Autodesk Fusion 360 part; units mm, degrees
(part 6 of 12)
  line L935 (-33.2373, 77.1244) -> (-33.2373, 72.1244)
  line L936 (-33.2373, 72.1244) -> (-28.9072, 69.6244)
  line L937 (-28.9072, 69.6244) -> (-24.577, 72.1244)
  line L938 (-24.577, 72.1244) -> (-24.577, 77.1244)
  line L939 (-24.577, 77.1244) -> (-28.9072, 79.6244)
  line L940 (-18.2469, 79.6244) -> (-22.577, 77.1244)
  line L941 (-22.577, 77.1244) -> (-22.577, 72.1244)
  line L942 (-22.577, 72.1244) -> (-18.2469, 69.6244)
  line L943 (-18.2469, 69.6244) -> (-13.9168, 72.1244)
  line L944 (-13.9168, 72.1244) -> (-13.9168, 77.1244)
  line L945 (-13.9168, 77.1244) -> (-18.2469, 79.6244)
  line L946 (-7.5866, 79.6244) -> (-11.9168, 77.1244)
  line L947 (-11.9168, 77.1244) -> (-11.9168, 72.1244)
  line L948 (-11.9168, 72.1244) -> (-7.5866, 69.6244)
  line L949 (-7.5866, 69.6244) -> (-3.2565, 72.1244)
  line L950 (-3.2565, 72.1244) -> (-3.2565, 77.1244)
  line L951 (-3.2565, 77.1244) -> (-7.5866, 79.6244)
  line L952 (3.0736, 79.6244) -> (-1.2565, 77.1244)
  line L953 (-1.2565, 77.1244) -> (-1.2565, 72.1244)
  line L954 (-1.2565, 72.1244) -> (3.0736, 69.6244)
  line L955 (3.0736, 69.6244) -> (7.4037, 72.1244)
  line L956 (7.4037, 72.1244) -> (7.4037, 77.1244)
  line L957 (7.4037, 77.1244) -> (3.0736, 79.6244)
  line L958 (13.7339, 79.6244) -> (9.4037, 77.1244)
  line L959 (9.4037, 77.1244) -> (9.4037, 72.1244)
  line L960 (9.4037, 72.1244) -> (13.7339, 69.6244)
  line L961 (13.7339, 69.6244) -> (18.064, 72.1244)
  line L962 (18.064, 72.1244) -> (18.064, 77.1244)
  line L963 (18.064, 77.1244) -> (13.7339, 79.6244)
  line L964 (24.3941, 79.6244) -> (20.064, 77.1244)
  line L965 (20.064, 77.1244) -> (20.064, 72.1244)
  line L966 (20.064, 72.1244) -> (24.3941, 69.6244)
  line L967 (24.3941, 69.6244) -> (28.7242, 72.1244)
  line L968 (28.7242, 72.1244) -> (28.7242, 77.1244)
  line L969 (28.7242, 77.1244) -> (24.3941, 79.6244)
  line L970 (35.0544, 79.6244) -> (30.7242, 77.1244)
  line L971 (30.7242, 77.1244) -> (30.7242, 72.1244)
  line L972 (30.7242, 72.1244) -> (35.0544, 69.6244)
  line L973 (35.0544, 69.6244) -> (39.3845, 72.1244)
  line L974 (39.3845, 72.1244) -> (39.3845, 77.1244)
  line L975 (39.3845, 77.1244) -> (35.0544, 79.6244)
  line L976 (45.7146, 79.6244) -> (41.3845, 77.1244)
  line L977 (41.3845, 77.1244) -> (41.3845, 72.1244)
  line L978 (41.3845, 72.1244) -> (45.7146, 69.6244)
  line L979 (45.7146, 69.6244) -> (50.0447, 72.1244)
  line L980 (50.0447, 72.1244) -> (50.0447, 77.1244)
  line L981 (50.0447, 77.1244) -> (45.7146, 79.6244)
  line L982 (56.3749, 79.6244) -> (52.0447, 77.1244)
  line L983 (52.0447, 77.1244) -> (52.0447, 72.1244)
  line L984 (52.0447, 72.1244) -> (56.3749, 69.6244)
  line L985 (56.3749, 69.6244) -> (60.705, 72.1244)
  line L986 (60.705, 72.1244) -> (60.705, 77.1244)
  line L987 (60.705, 77.1244) -> (56.3749, 79.6244)
  line L988 (-151.5001, 88.8564) -> (-155.8302, 86.3564)
  line L989 (-155.8302, 86.3564) -> (-155.8302, 81.3564)
  line L990 (-155.8302, 81.3564) -> (-151.5001, 78.8564)
  line L991 (-151.5001, 78.8564) -> (-147.17, 81.3564)
  line L992 (-147.17, 81.3564) -> (-147.17, 86.3564)
  line L993 (-147.17, 86.3564) -> (-151.5001, 88.8564)
  line L994 (-140.8398, 88.8564) -> (-145.17, 86.3564)
  line L995 (-145.17, 86.3564) -> (-145.17, 81.3564)
  line L996 (-145.17, 81.3564) -> (-140.8398, 78.8564)
  line L997 (-140.8398, 78.8564) -> (-136.5097, 81.3564)
  line L998 (-136.5097, 81.3564) -> (-136.5097, 86.3564)
  line L999 (-136.5097, 86.3564) -> (-140.8398, 88.8564)
  line L1000 (-130.1796, 88.8564) -> (-134.5097, 86.3564)
  line L1001 (-134.5097, 86.3564) -> (-134.5097, 81.3564)
  line L1002 (-134.5097, 81.3564) -> (-130.1796, 78.8564)
  line L1003 (-130.1796, 78.8564) -> (-125.8494, 81.3564)
  line L1004 (-125.8494, 81.3564) -> (-125.8494, 86.3564)
  line L1005 (-125.8494, 86.3564) -> (-130.1796, 88.8564)
  line L1006 (-119.5193, 88.8564) -> (-123.8494, 86.3564)
  line L1007 (-123.8494, 86.3564) -> (-123.8494, 81.3564)
  line L1008 (-123.8494, 81.3564) -> (-119.5193, 78.8564)
  line L1009 (-119.5193, 78.8564) -> (-115.1892, 81.3564)
  line L1010 (-115.1892, 81.3564) -> (-115.1892, 86.3564)
  line L1011 (-115.1892, 86.3564) -> (-119.5193, 88.8564)
  line L1012 (-108.8591, 88.8564) -> (-113.1892, 86.3564)
  line L1013 (-113.1892, 86.3564) -> (-113.1892, 81.3564)
  line L1014 (-113.1892, 81.3564) -> (-108.8591, 78.8564)
  line L1015 (-108.8591, 78.8564) -> (-104.5289, 81.3564)
  line L1016 (-104.5289, 81.3564) -> (-104.5289, 86.3564)
  line L1017 (-104.5289, 86.3564) -> (-108.8591, 88.8564)
  line L1018 (-98.1988, 88.8564) -> (-102.5289, 86.3564)
  line L1019 (-102.5289, 86.3564) -> (-102.5289, 81.3564)
  line L1020 (-102.5289, 81.3564) -> (-98.1988, 78.8564)
  line L1021 (-98.1988, 78.8564) -> (-93.8687, 81.3564)
  line L1022 (-93.8687, 81.3564) -> (-93.8687, 86.3564)
  line L1023 (-93.8687, 86.3564) -> (-98.1988, 88.8564)
  line L1024 (-87.5386, 88.8564) -> (-91.8687, 86.3564)
  line L1025 (-91.8687, 86.3564) -> (-91.8687, 81.3564)
  line L1026 (-91.8687, 81.3564) -> (-87.5386, 78.8564)
  line L1027 (-87.5386, 78.8564) -> (-83.2084, 81.3564)
  line L1028 (-83.2084, 81.3564) -> (-83.2084, 86.3564)
  line L1029 (-83.2084, 86.3564) -> (-87.5386, 88.8564)
  line L1030 (-76.8783, 88.8564) -> (-81.2084, 86.3564)
  line L1031 (-81.2084, 86.3564) -> (-81.2084, 81.3564)
  line L1032 (-81.2084, 81.3564) -> (-76.8783, 78.8564)
  line L1033 (-76.8783, 78.8564) -> (-72.5482, 81.3564)
  line L1034 (-72.5482, 81.3564) -> (-72.5482, 86.3564)
  line L1035 (-72.5482, 86.3564) -> (-76.8783, 88.8564)
  line L1036 (-66.218, 88.8564) -> (-70.5482, 86.3564)
  line L1037 (-70.5482, 86.3564) -> (-70.5482, 81.3564)
  line L1038 (-70.5482, 81.3564) -> (-66.218, 78.8564)
  line L1039 (-66.218, 78.8564) -> (-61.8879, 81.3564)
  line L1040 (-61.8879, 81.3564) -> (-61.8879, 86.3564)
  line L1041 (-61.8879, 86.3564) -> (-66.218, 88.8564)
  line L1042 (-55.5578, 88.8564) -> (-59.8879, 86.3564)
  line L1043 (-59.8879, 86.3564) -> (-59.8879, 81.3564)
  line L1044 (-59.8879, 81.3564) -> (-55.5578, 78.8564)
  line L1045 (-55.5578, 78.8564) -> (-51.2277, 81.3564)
  line L1046 (-51.2277, 81.3564) -> (-51.2277, 86.3564)
  line L1047 (-51.2277, 86.3564) -> (-55.5578, 88.8564)
  line L1048 (-44.8975, 88.8564) -> (-49.2277, 86.3564)
  line L1049 (-49.2277, 86.3564) -> (-49.2277, 81.3564)
  line L1050 (-49.2277, 81.3564) -> (-44.8975, 78.8564)
  line L1051 (-44.8975, 78.8564) -> (-40.5674, 81.3564)
  line L1052 (-40.5674, 81.3564) -> (-40.5674, 86.3564)
  line L1053 (-40.5674, 86.3564) -> (-44.8975, 88.8564)
  line L1054 (-34.2373, 88.8564) -> (-38.5674, 86.3564)
  line L1055 (-38.5674, 86.3564) -> (-38.5674, 81.3564)
  line L1056 (-38.5674, 81.3564) -> (-34.2373, 78.8564)
  line L1057 (-34.2373, 78.8564) -> (-29.9072, 81.3564)
  line L1058 (-29.9072, 81.3564) -> (-29.9072, 86.3564)
  line L1059 (-29.9072, 86.3564) -> (-34.2373, 88.8564)
  line L1060 (-23.577, 88.8564) -> (-27.9072, 86.3564)
  line L1061 (-27.9072, 86.3564) -> (-27.9072, 81.3564)
  line L1062 (-27.9072, 81.3564) -> (-23.577, 78.8564)
  line L1063 (-23.577, 78.8564) -> (-19.2469, 81.3564)
  line L1064 (-19.2469, 81.3564) -> (-19.2469, 86.3564)
  line L1065 (-19.2469, 86.3564) -> (-23.577, 88.8564)
  line L1066 (-12.9168, 88.8564) -> (-17.2469, 86.3564)
  line L1067 (-17.2469, 86.3564) -> (-17.2469, 81.3564)
  line L1068 (-17.2469, 81.3564) -> (-12.9168, 78.8564)
  line L1069 (-12.9168, 78.8564) -> (-8.5866, 81.3564)
  line L1070 (-8.5866, 81.3564) -> (-8.5866, 86.3564)
  line L1071 (-8.5866, 86.3564) -> (-12.9168, 88.8564)
  line L1072 (-2.2565, 88.8564) -> (-6.5866, 86.3564)
  line L1073 (-6.5866, 86.3564) -> (-6.5866, 81.3564)
  line L1074 (-6.5866, 81.3564) -> (-2.2565, 78.8564)
  line L1075 (-2.2565, 78.8564) -> (2.0736, 81.3564)
  line L1076 (2.0736, 81.3564) -> (2.0736, 86.3564)
  line L1077 (2.0736, 86.3564) -> (-2.2565, 88.8564)
  line L1078 (8.4037, 88.8564) -> (4.0736, 86.3564)
  line L1079 (4.0736, 86.3564) -> (4.0736, 81.3564)
  line L1080 (4.0736, 81.3564) -> (8.4037, 78.8564)
  line L1081 (8.4037, 78.8564) -> (12.7339, 81.3564)
  line L1082 (12.7339, 81.3564) -> (12.7339, 86.3564)
  line L1083 (12.7339, 86.3564) -> (8.4037, 88.8564)
  line L1084 (19.064, 88.8564) -> (14.7339, 86.3564)
  line L1085 (14.7339, 86.3564) -> (14.7339, 81.3564)
  line L1086 (14.7339, 81.3564) -> (19.064, 78.8564)
  line L1087 (19.064, 78.8564) -> (23.3941, 81.3564)
  line L1088 (23.3941, 81.3564) -> (23.3941, 86.3564)
  line L1089 (23.3941, 86.3564) -> (19.064, 88.8564)
  line L1090 (29.7242, 88.8564) -> (25.3941, 86.3564)
  line L1091 (25.3941, 86.3564) -> (25.3941, 81.3564)
  line L1092 (25.3941, 81.3564) -> (29.7242, 78.8564)
  line L1093 (29.7242, 78.8564) -> (34.0544, 81.3564)
  line L1094 (34.0544, 81.3564) -> (34.0544, 86.3564)
  line L1095 (34.0544, 86.3564) -> (29.7242, 88.8564)
  line L1096 (40.3845, 88.8564) -> (36.0544, 86.3564)
  line L1097 (36.0544, 86.3564) -> (36.0544, 81.3564)
  line L1098 (36.0544, 81.3564) -> (40.3845, 78.8564)
  line L1099 (40.3845, 78.8564) -> (44.7146, 81.3564)
  line L1100 (44.7146, 81.3564) -> (44.7146, 86.3564)
  line L1101 (44.7146, 86.3564) -> (40.3845, 88.8564)
  line L1102 (51.0447, 88.8564) -> (46.7146, 86.3564)
  line L1103 (46.7146, 86.3564) -> (46.7146, 81.3564)
  line L1104 (46.7146, 81.3564) -> (51.0447, 78.8564)
  line L1105 (51.0447, 78.8564) -> (55.3749, 81.3564)
  line L1106 (55.3749, 81.3564) -> (55.3749, 86.3564)
  line L1107 (55.3749, 86.3564) -> (51.0447, 88.8564)
  line L1108 (61.705, 88.8564) -> (57.3749, 86.3564)
  line L1109 (57.3749, 86.3564) -> (57.3749, 81.3564)
  line L1110 (57.3749, 81.3564) -> (61.705, 78.8564)
  line L1111 (61.705, 78.8564) -> (66.0351, 81.3564)
  line L1112 (66.0351, 81.3564) -> (66.0351, 86.3564)
  line L1113 (66.0351, 86.3564) -> (61.705, 88.8564)
  line L1114 (-146.17, 98.0885) -> (-150.5001, 95.5885)
  line L1115 (-150.5001, 95.5885) -> (-150.5001, 90.5885)
  line L1116 (-150.5001, 90.5885) -> (-146.17, 88.0885)
  line L1117 (-146.17, 88.0885) -> (-141.8398, 90.5885)
  line L1118 (-141.8398, 90.5885) -> (-141.8398, 95.5885)
  line L1119 (-141.8398, 95.5885) -> (-146.17, 98.0885)
  line L1120 (-135.5097, 98.0885) -> (-139.8398, 95.5885)
  line L1121 (-139.8398, 95.5885) -> (-139.8398, 90.5885)
  line L1122 (-139.8398, 90.5885) -> (-135.5097, 88.0885)
  line L1123 (-135.5097, 88.0885) -> (-131.1796, 90.5885)
  line L1124 (-131.1796, 90.5885) -> (-131.1796, 95.5885)
  line L1125 (-131.1796, 95.5885) -> (-135.5097, 98.0885)
  line L1126 (-124.8494, 98.0885) -> (-129.1796, 95.5885)
  line L1127 (-129.1796, 95.5885) -> (-129.1796, 90.5885)
  line L1128 (-129.1796, 90.5885) -> (-124.8494, 88.0885)
  line L1129 (-124.8494, 88.0885) -> (-120.5193, 90.5885)
  line L1130 (-120.5193, 90.5885) -> (-120.5193, 95.5885)
  line L1131 (-120.5193, 95.5885) -> (-124.8494, 98.0885)
  line L1132 (-114.1892, 98.0885) -> (-118.5193, 95.5885)
  line L1133 (-118.5193, 95.5885) -> (-118.5193, 90.5885)
  line L1134 (-118.5193, 90.5885) -> (-114.1892, 88.0885)
  line L1135 (-114.1892, 88.0885) -> (-109.8591, 90.5885)
  line L1136 (-109.8591, 90.5885) -> (-109.8591, 95.5885)
  line L1137 (-109.8591, 95.5885) -> (-114.1892, 98.0885)
  line L1138 (-103.5289, 98.0885) -> (-107.8591, 95.5885)
  line L1139 (-107.8591, 95.5885) -> (-107.8591, 90.5885)
  line L1140 (-107.8591, 90.5885) -> (-103.5289, 88.0885)
  line L1141 (-103.5289, 88.0885) -> (-99.1988, 90.5885)
  line L1142 (-99.1988, 90.5885) -> (-99.1988, 95.5885)
  line L1143 (-99.1988, 95.5885) -> (-103.5289, 98.0885)
  line L1144 (-92.8687, 98.0885) -> (-97.1988, 95.5885)
  line L1145 (-97.1988, 95.5885) -> (-97.1988, 90.5885)
  line L1146 (-97.1988, 90.5885) -> (-92.8687, 88.0885)
  line L1147 (-92.8687, 88.0885) -> (-88.5386, 90.5885)
  line L1148 (-88.5386, 90.5885) -> (-88.5386, 95.5885)
  line L1149 (-88.5386, 95.5885) -> (-92.8687, 98.0885)
  line L1150 (-82.2084, 98.0885) -> (-86.5386, 95.5885)
  line L1151 (-86.5386, 95.5885) -> (-86.5386, 90.5885)
  line L1152 (-86.5386, 90.5885) -> (-82.2084, 88.0885)
  line L1153 (-82.2084, 88.0885) -> (-77.8783, 90.5885)
  line L1154 (-77.8783, 90.5885) -> (-77.8783, 95.5885)
  line L1155 (-77.8783, 95.5885) -> (-82.2084, 98.0885)
  line L1156 (-71.5482, 98.0885) -> (-75.8783, 95.5885)
  line L1157 (-75.8783, 95.5885) -> (-75.8783, 90.5885)
  line L1158 (-75.8783, 90.5885) -> (-71.5482, 88.0885)
  line L1159 (-71.5482, 88.0885) -> (-67.218, 90.5885)
  line L1160 (-67.218, 90.5885) -> (-67.218, 95.5885)
  line L1161 (-67.218, 95.5885) -> (-71.5482, 98.0885)
  line L1162 (-60.8879, 98.0885) -> (-65.218, 95.5885)
  line L1163 (-65.218, 95.5885) -> (-65.218, 90.5885)
  line L1164 (-65.218, 90.5885) -> (-60.8879, 88.0885)
  line L1165 (-60.8879, 88.0885) -> (-56.5578, 90.5885)
  line L1166 (-56.5578, 90.5885) -> (-56.5578, 95.5885)
  line L1167 (-56.5578, 95.5885) -> (-60.8879, 98.0885)
  line L1168 (-50.2277, 98.0885) -> (-54.5578, 95.5885)
  line L1169 (-54.5578, 95.5885) -> (-54.5578, 90.5885)
  line L1170 (-54.5578, 90.5885) -> (-50.2277, 88.0885)
  line L1171 (-50.2277, 88.0885) -> (-45.8975, 90.5885)
  line L1172 (-45.8975, 90.5885) -> (-45.8975, 95.5885)
  line L1173 (-45.8975, 95.5885) -> (-50.2277, 98.0885)
  line L1174 (-39.5674, 98.0885) -> (-43.8975, 95.5885)
  line L1175 (-43.8975, 95.5885) -> (-43.8975, 90.5885)
  line L1176 (-43.8975, 90.5885) -> (-39.5674, 88.0885)
  line L1177 (-39.5674, 88.0885) -> (-35.2373, 90.5885)
  line L1178 (-35.2373, 90.5885) -> (-35.2373, 95.5885)
  line L1179 (-35.2373, 95.5885) -> (-39.5674, 98.0885)
  line L1180 (-28.9072, 98.0885) -> (-33.2373, 95.5885)
  line L1181 (-33.2373, 95.5885) -> (-33.2373, 90.5885)
  line L1182 (-33.2373, 90.5885) -> (-28.9072, 88.0885)
  line L1183 (-28.9072, 88.0885) -> (-24.577, 90.5885)
  line L1184 (-24.577, 90.5885) -> (-24.577, 95.5885)
  line L1185 (-24.577, 95.5885) -> (-28.9072, 98.0885)
  line L1186 (-18.2469, 98.0885) -> (-22.577, 95.5885)
  line L1187 (-22.577, 95.5885) -> (-22.577, 90.5885)
  line L1188 (-22.577, 90.5885) -> (-18.2469, 88.0885)
  line L1189 (-18.2469, 88.0885) -> (-13.9168, 90.5885)
  line L1190 (-13.9168, 90.5885) -> (-13.9168, 95.5885)
  line L1191 (-13.9168, 95.5885) -> (-18.2469, 98.0885)
  line L1192 (-7.5866, 98.0885) -> (-11.9168, 95.5885)
  line L1193 (-11.9168, 95.5885) -> (-11.9168, 90.5885)
  line L1194 (-11.9168, 90.5885) -> (-7.5866, 88.0885)
  line L1195 (-7.5866, 88.0885) -> (-3.2565, 90.5885)
  line L1196 (-3.2565, 90.5885) -> (-3.2565, 95.5885)
  line L1197 (-3.2565, 95.5885) -> (-7.5866, 98.0885)
  line L1198 (3.0736, 98.0885) -> (-1.2565, 95.5885)
  line L1199 (-1.2565, 95.5885) -> (-1.2565, 90.5885)
  line L1200 (-1.2565, 90.5885) -> (3.0736, 88.0885)
  line L1201 (3.0736, 88.0885) -> (7.4037, 90.5885)
  line L1202 (7.4037, 90.5885) -> (7.4037, 95.5885)
  line L1203 (7.4037, 95.5885) -> (3.0736, 98.0885)
  line L1204 (13.7339, 98.0885) -> (9.4037, 95.5885)
  line L1205 (9.4037, 95.5885) -> (9.4037, 90.5885)
  line L1206 (9.4037, 90.5885) -> (13.7339, 88.0885)
  line L1207 (13.7339, 88.0885) -> (18.064, 90.5885)
  line L1208 (18.064, 90.5885) -> (18.064, 95.5885)
  line L1209 (18.064, 95.5885) -> (13.7339, 98.0885)
  line L1210 (24.3941, 98.0885) -> (20.064, 95.5885)
  line L1211 (20.064, 95.5885) -> (20.064, 90.5885)
  line L1212 (20.064, 90.5885) -> (24.3941, 88.0885)
  line L1213 (24.3941, 88.0885) -> (28.7242, 90.5885)
  line L1214 (28.7242, 90.5885) -> (28.7242, 95.5885)
  line L1215 (28.7242, 95.5885) -> (24.3941, 98.0885)
  line L1216 (35.0544, 98.0885) -> (30.7242, 95.5885)
  line L1217 (30.7242, 95.5885) -> (30.7242, 90.5885)
  line L1218 (30.7242, 90.5885) -> (35.0544, 88.0885)
  line L1219 (35.0544, 88.0885) -> (39.3845, 90.5885)
  line L1220 (39.3845, 90.5885) -> (39.3845, 95.5885)
  line L1221 (39.3845, 95.5885) -> (35.0544, 98.0885)
  line L1222 (45.7146, 98.0885) -> (41.3845, 95.5885)
  line L1223 (41.3845, 95.5885) -> (41.3845, 90.5885)
  line L1224 (41.3845, 90.5885) -> (45.7146, 88.0885)
  line L1225 (45.7146, 88.0885) -> (50.0447, 90.5885)
  line L1226 (50.0447, 90.5885) -> (50.0447, 95.5885)
  line L1227 (50.0447, 95.5885) -> (45.7146, 98.0885)
  line L1228 (56.3749, 98.0885) -> (52.0447, 95.5885)
  line L1229 (52.0447, 95.5885) -> (52.0447, 90.5885)
  line L1230 (52.0447, 90.5885) -> (56.3749, 88.0885)
  line L1231 (56.3749, 88.0885) -> (60.705, 90.5885)
  line L1232 (60.705, 90.5885) -> (60.705, 95.5885)
  line L1233 (60.705, 95.5885) -> (56.3749, 98.0885)
  line L1234 (-151.5001, 107.3205) -> (-155.8302, 104.8205)
  line L1235 (-155.8302, 104.8205) -> (-155.8302, 99.8205)
  line L1236 (-155.8302, 99.8205) -> (-151.5001, 97.3205)
  line L1237 (-151.5001, 97.3205) -> (-147.17, 99.8205)
  line L1238 (-147.17, 99.8205) -> (-147.17, 104.8205)
  line L1239 (-147.17, 104.8205) -> (-151.5001, 107.3205)
  line L1240 (-140.8398, 107.3205) -> (-145.17, 104.8205)
  line L1241 (-145.17, 104.8205) -> (-145.17, 99.8205)
  line L1242 (-145.17, 99.8205) -> (-140.8398, 97.3205)
  line L1243 (-140.8398, 97.3205) -> (-136.5097, 99.8205)
  line L1244 (-136.5097, 99.8205) -> (-136.5097, 104.8205)
  line L1245 (-136.5097, 104.8205) -> (-140.8398, 107.3205)
  line L1246 (-130.1796, 107.3205) -> (-134.5097, 104.8205)
  line L1247 (-134.5097, 104.8205) -> (-134.5097, 99.8205)
  line L1248 (-134.5097, 99.8205) -> (-130.1796, 97.3205)
  line L1249 (-130.1796, 97.3205) -> (-125.8494, 99.8205)
  line L1250 (-125.8494, 99.8205) -> (-125.8494, 104.8205)
  line L1251 (-125.8494, 104.8205) -> (-130.1796, 107.3205)
  line L1252 (-119.5193, 107.3205) -> (-123.8494, 104.8205)
  line L1253 (-123.8494, 104.8205) -> (-123.8494, 99.8205)
  line L1254 (-123.8494, 99.8205) -> (-119.5193, 97.3205)
  line L1255 (-119.5193, 97.3205) -> (-115.1892, 99.8205)
  line L1256 (-115.1892, 99.8205) -> (-115.1892, 104.8205)
  line L1257 (-115.1892, 104.8205) -> (-119.5193, 107.3205)
  line L1258 (-108.8591, 107.3205) -> (-113.1892, 104.8205)
  line L1259 (-113.1892, 104.8205) -> (-113.1892, 99.8205)
  line L1260 (-113.1892, 99.8205) -> (-108.8591, 97.3205)
  line L1261 (-108.8591, 97.3205) -> (-104.5289, 99.8205)
  line L1262 (-104.5289, 99.8205) -> (-104.5289, 104.8205)
  line L1263 (-104.5289, 104.8205) -> (-108.8591, 107.3205)
  line L1264 (-98.1988, 107.3205) -> (-102.5289, 104.8205)
  line L1265 (-102.5289, 104.8205) -> (-102.5289, 99.8205)
  line L1266 (-102.5289, 99.8205) -> (-98.1988, 97.3205)
  line L1267 (-98.1988, 97.3205) -> (-93.8687, 99.8205)
  line L1268 (-93.8687, 99.8205) -> (-93.8687, 104.8205)
  line L1269 (-93.8687, 104.8205) -> (-98.1988, 107.3205)
  line L1270 (-87.5386, 107.3205) -> (-91.8687, 104.8205)
  line L1271 (-91.8687, 104.8205) -> (-91.8687, 99.8205)
  line L1272 (-91.8687, 99.8205) -> (-87.5386, 97.3205)
  line L1273 (-87.5386, 97.3205) -> (-83.2084, 99.8205)
  line L1274 (-83.2084, 99.8205) -> (-83.2084, 104.8205)
  line L1275 (-83.2084, 104.8205) -> (-87.5386, 107.3205)
  line L1276 (-76.8783, 107.3205) -> (-81.2084, 104.8205)
  line L1277 (-81.2084, 104.8205) -> (-81.2084, 99.8205)
  line L1278 (-81.2084, 99.8205) -> (-76.8783, 97.3205)
  line L1279 (-76.8783, 97.3205) -> (-72.5482, 99.8205)
  line L1280 (-72.5482, 99.8205) -> (-72.5482, 104.8205)
  line L1281 (-72.5482, 104.8205) -> (-76.8783, 107.3205)
  line L1282 (-66.218, 107.3205) -> (-70.5482, 104.8205)
  line L1283 (-70.5482, 104.8205) -> (-70.5482, 99.8205)
  line L1284 (-70.5482, 99.8205) -> (-66.218, 97.3205)
  line L1285 (-66.218, 97.3205) -> (-61.8879, 99.8205)
  line L1286 (-61.8879, 99.8205) -> (-61.8879, 104.8205)
  line L1287 (-61.8879, 104.8205) -> (-66.218, 107.3205)
  line L1288 (-55.5578, 107.3205) -> (-59.8879, 104.8205)
  line L1289 (-59.8879, 104.8205) -> (-59.8879, 99.8205)
  line L1290 (-59.8879, 99.8205) -> (-55.5578, 97.3205)
  line L1291 (-55.5578, 97.3205) -> (-51.2277, 99.8205)
  line L1292 (-51.2277, 99.8205) -> (-51.2277, 104.8205)
  line L1293 (-51.2277, 104.8205) -> (-55.5578, 107.3205)
  line L1294 (-44.8975, 107.3205) -> (-49.2277, 104.8205)
  line L1295 (-49.2277, 104.8205) -> (-49.2277, 99.8205)
  line L1296 (-49.2277, 99.8205) -> (-44.8975, 97.3205)
  line L1297 (-44.8975, 97.3205) -> (-40.5674, 99.8205)
  line L1298 (-40.5674, 99.8205) -> (-40.5674, 104.8205)
  line L1299 (-40.5674, 104.8205) -> (-44.8975, 107.3205)
  line L1300 (-34.2373, 107.3205) -> (-38.5674, 104.8205)
  line L1301 (-38.5674, 104.8205) -> (-38.5674, 99.8205)
  line L1302 (-38.5674, 99.8205) -> (-34.2373, 97.3205)
  line L1303 (-34.2373, 97.3205) -> (-29.9072, 99.8205)
  line L1304 (-29.9072, 99.8205) -> (-29.9072, 104.8205)
  line L1305 (-29.9072, 104.8205) -> (-34.2373, 107.3205)
  line L1306 (-23.577, 107.3205) -> (-27.9072, 104.8205)
  line L1307 (-27.9072, 104.8205) -> (-27.9072, 99.8205)
  line L1308 (-27.9072, 99.8205) -> (-23.577, 97.3205)
  line L1309 (-23.577, 97.3205) -> (-19.2469, 99.8205)
  line L1310 (-19.2469, 99.8205) -> (-19.2469, 104.8205)
  line L1311 (-19.2469, 104.8205) -> (-23.577, 107.3205)
  line L1312 (-12.9168, 107.3205) -> (-17.2469, 104.8205)
  line L1313 (-17.2469, 104.8205) -> (-17.2469, 99.8205)
  line L1314 (-17.2469, 99.8205) -> (-12.9168, 97.3205)
  line L1315 (-12.9168, 97.3205) -> (-8.5866, 99.8205)
  line L1316 (-8.5866, 99.8205) -> (-8.5866, 104.8205)
  line L1317 (-8.5866, 104.8205) -> (-12.9168, 107.3205)
  line L1318 (-2.2565, 107.3205) -> (-6.5866, 104.8205)
  line L1319 (-6.5866, 104.8205) -> (-6.5866, 99.8205)
  line L1320 (-6.5866, 99.8205) -> (-2.2565, 97.3205)
  line L1321 (-2.2565, 97.3205) -> (2.0736, 99.8205)
  line L1322 (2.0736, 99.8205) -> (2.0736, 104.8205)
  line L1323 (2.0736, 104.8205) -> (-2.2565, 107.3205)
  line L1324 (8.4037, 107.3205) -> (4.0736, 104.8205)
  line L1325 (4.0736, 104.8205) -> (4.0736, 99.8205)
  line L1326 (4.0736, 99.8205) -> (8.4037, 97.3205)
  line L1327 (8.4037, 97.3205) -> (12.7339, 99.8205)
  line L1328 (12.7339, 99.8205) -> (12.7339, 104.8205)
  line L1329 (12.7339, 104.8205) -> (8.4037, 107.3205)
  line L1330 (19.064, 107.3205) -> (14.7339, 104.8205)
  line L1331 (14.7339, 104.8205) -> (14.7339, 99.8205)
  line L1332 (14.7339, 99.8205) -> (19.064, 97.3205)
  line L1333 (19.064, 97.3205) -> (23.3941, 99.8205)
  line L1334 (23.3941, 99.8205) -> (23.3941, 104.8205)
  line L1335 (23.3941, 104.8205) -> (19.064, 107.3205)
  line L1336 (29.7242, 107.3205) -> (25.3941, 104.8205)
  line L1337 (25.3941, 104.8205) -> (25.3941, 99.8205)
  line L1338 (25.3941, 99.8205) -> (29.7242, 97.3205)
  line L1339 (29.7242, 97.3205) -> (34.0544, 99.8205)
  line L1340 (34.0544, 99.8205) -> (34.0544, 104.8205)
  line L1341 (34.0544, 104.8205) -> (29.7242, 107.3205)
  line L1342 (40.3845, 107.3205) -> (36.0544, 104.8205)
  line L1343 (36.0544, 104.8205) -> (36.0544, 99.8205)
  line L1344 (36.0544, 99.8205) -> (40.3845, 97.3205)
  line L1345 (40.3845, 97.3205) -> (44.7146, 99.8205)
  line L1346 (44.7146, 99.8205) -> (44.7146, 104.8205)
  line L1347 (44.7146, 104.8205) -> (40.3845, 107.3205)
  line L1348 (51.0447, 107.3205) -> (46.7146, 104.8205)
  line L1349 (46.7146, 104.8205) -> (46.7146, 99.8205)
  line L1350 (46.7146, 99.8205) -> (51.0447, 97.3205)
  line L1351 (51.0447, 97.3205) -> (55.3749, 99.8205)
  line L1352 (55.3749, 99.8205) -> (55.3749, 104.8205)
  line L1353 (55.3749, 104.8205) -> (51.0447, 107.3205)
  line L1354 (61.705, 107.3205) -> (57.3749, 104.8205)
  line L1355 (57.3749, 104.8205) -> (57.3749, 99.8205)
  line L1356 (57.3749, 99.8205) -> (61.705, 97.3205)
  line L1357 (61.705, 97.3205) -> (66.0351, 99.8205)
  line L1358 (66.0351, 99.8205) -> (66.0351, 104.8205)
  line L1359 (66.0351, 104.8205) -> (61.705, 107.3205)
  line L1360 (-146.17, 116.5526) -> (-150.5001, 114.0526)
  line L1361 (-150.5001, 114.0526) -> (-150.5001, 109.0526)
  line L1362 (-150.5001, 109.0526) -> (-146.17, 106.5526)
  line L1363 (-146.17, 106.5526) -> (-141.8398, 109.0526)
  line L1364 (-141.8398, 109.0526) -> (-141.8398, 114.0526)
  line L1365 (-141.8398, 114.0526) -> (-146.17, 116.5526)
  line L1366 (-135.5097, 116.5526) -> (-139.8398, 114.0526)
  line L1367 (-139.8398, 114.0526) -> (-139.8398, 109.0526)
  line L1368 (-139.8398, 109.0526) -> (-135.5097, 106.5526)
  line L1369 (-135.5097, 106.5526) -> (-131.1796, 109.0526)
  line L1370 (-131.1796, 109.0526) -> (-131.1796, 114.0526)
  line L1371 (-131.1796, 114.0526) -> (-135.5097, 116.5526)
  line L1372 (-124.8494, 116.5526) -> (-129.1796, 114.0526)
  line L1373 (-129.1796, 114.0526) -> (-129.1796, 109.0526)
  line L1374 (-129.1796, 109.0526) -> (-124.8494, 106.5526)
  line L1375 (-124.8494, 106.5526) -> (-120.5193, 109.0526)
  line L1376 (-120.5193, 109.0526) -> (-120.5193, 114.0526)
  line L1377 (-120.5193, 114.0526) -> (-124.8494, 116.5526)
  line L1378 (-114.1892, 116.5526) -> (-118.5193, 114.0526)
  line L1379 (-118.5193, 114.0526) -> (-118.5193, 109.0526)
  line L1380 (-118.5193, 109.0526) -> (-114.1892, 106.5526)
  line L1381 (-114.1892, 106.5526) -> (-109.8591, 109.0526)
  line L1382 (-109.8591, 109.0526) -> (-109.8591, 114.0526)
  line L1383 (-109.8591, 114.0526) -> (-114.1892, 116.5526)
  line L1384 (-103.5289, 116.5526) -> (-107.8591, 114.0526)
  line L1385 (-107.8591, 114.0526) -> (-107.8591, 109.0526)
  line L1386 (-107.8591, 109.0526) -> (-103.5289, 106.5526)
  line L1387 (-103.5289, 106.5526) -> (-99.1988, 109.0526)
  line L1388 (-99.1988, 109.0526) -> (-99.1988, 114.0526)
  line L1389 (-99.1988, 114.0526) -> (-103.5289, 116.5526)
  line L1390 (-92.8687, 116.5526) -> (-97.1988, 114.0526)
  line L1391 (-97.1988, 114.0526) -> (-97.1988, 109.0526)
  line L1392 (-97.1988, 109.0526) -> (-92.8687, 106.5526)
  line L1393 (-92.8687, 106.5526) -> (-88.5386, 109.0526)
  line L1394 (-88.5386, 109.0526) -> (-88.5386, 114.0526)
  line L1395 (-88.5386, 114.0526) -> (-92.8687, 116.5526)
  line L1396 (-82.2084, 116.5526) -> (-86.5386, 114.0526)
  line L1397 (-86.5386, 114.0526) -> (-86.5386, 109.0526)
  line L1398 (-86.5386, 109.0526) -> (-82.2084, 106.5526)
  line L1399 (-82.2084, 106.5526) -> (-77.8783, 109.0526)
  line L1400 (-77.8783, 109.0526) -> (-77.8783, 114.0526)
  line L1401 (-77.8783, 114.0526) -> (-82.2084, 116.5526)
  line L1402 (-71.5482, 116.5526) -> (-75.8783, 114.0526)
  line L1403 (-75.8783, 114.0526) -> (-75.8783, 109.0526)
  line L1404 (-75.8783, 109.0526) -> (-71.5482, 106.5526)
  line L1405 (-71.5482, 106.5526) -> (-67.218, 109.0526)
  line L1406 (-67.218, 109.0526) -> (-67.218, 114.0526)
  line L1407 (-67.218, 114.0526) -> (-71.5482, 116.5526)
  line L1408 (-60.8879, 116.5526) -> (-65.218, 114.0526)
  line L1409 (-65.218, 114.0526) -> (-65.218, 109.0526)
  line L1410 (-65.218, 109.0526) -> (-60.8879, 106.5526)
  line L1411 (-60.8879, 106.5526) -> (-56.5578, 109.0526)
  line L1412 (-56.5578, 109.0526) -> (-56.5578, 114.0526)
  line L1413 (-56.5578, 114.0526) -> (-60.8879, 116.5526)
  line L1414 (-50.2277, 116.5526) -> (-54.5578, 114.0526)
  line L1415 (-54.5578, 114.0526) -> (-54.5578, 109.0526)
  line L1416 (-54.5578, 109.0526) -> (-50.2277, 106.5526)
  line L1417 (-50.2277, 106.5526) -> (-45.8975, 109.0526)
  line L1418 (-45.8975, 109.0526) -> (-45.8975, 114.0526)
  line L1419 (-45.8975, 114.0526) -> (-50.2277, 116.5526)
  line L1420 (-39.5674, 116.5526) -> (-43.8975, 114.0526)
  line L1421 (-43.8975, 114.0526) -> (-43.8975, 109.0526)
  line L1422 (-43.8975, 109.0526) -> (-39.5674, 106.5526)
  line L1423 (-39.5674, 106.5526) -> (-35.2373, 109.0526)
  line L1424 (-35.2373, 109.0526) -> (-35.2373, 114.0526)
  line L1425 (-35.2373, 114.0526) -> (-39.5674, 116.5526)
  line L1426 (-28.9072, 116.5526) -> (-33.2373, 114.0526)
  line L1427 (-33.2373, 114.0526) -> (-33.2373, 109.0526)
  line L1428 (-33.2373, 109.0526) -> (-28.9072, 106.5526)
  line L1429 (-28.9072, 106.5526) -> (-24.577, 109.0526)
  line L1430 (-24.577, 109.0526) -> (-24.577, 114.0526)
  line L1431 (-24.577, 114.0526) -> (-28.9072, 116.5526)
  line L1432 (-18.2469, 116.5526) -> (-22.577, 114.0526)
  line L1433 (-22.577, 114.0526) -> (-22.577, 109.0526)
  line L1434 (-22.577, 109.0526) -> (-18.2469, 106.5526)
  line L1435 (-18.2469, 106.5526) -> (-13.9168, 109.0526)
  line L1436 (-13.9168, 109.0526) -> (-13.9168, 114.0526)
  line L1437 (-13.9168, 114.0526) -> (-18.2469, 116.5526)
  line L1438 (-7.5866, 116.5526) -> (-11.9168, 114.0526)
  line L1439 (-11.9168, 114.0526) -> (-11.9168, 109.0526)
  line L1440 (-11.9168, 109.0526) -> (-7.5866, 106.5526)
  line L1441 (-7.5866, 106.5526) -> (-3.2565, 109.0526)
  line L1442 (-3.2565, 109.0526) -> (-3.2565, 114.0526)
  line L1443 (-3.2565, 114.0526) -> (-7.5866, 116.5526)
  line L1444 (3.0736, 116.5526) -> (-1.2565, 114.0526)
  line L1445 (-1.2565, 114.0526) -> (-1.2565, 109.0526)
  line L1446 (-1.2565, 109.0526) -> (3.0736, 106.5526)
  line L1447 (3.0736, 106.5526) -> (7.4037, 109.0526)
  line L1448 (7.4037, 109.0526) -> (7.4037, 114.0526)
  line L1449 (7.4037, 114.0526) -> (3.0736, 116.5526)
  line L1450 (13.7339, 116.5526) -> (9.4037, 114.0526)
  line L1451 (9.4037, 114.0526) -> (9.4037, 109.0526)
  line L1452 (9.4037, 109.0526) -> (13.7339, 106.5526)
  line L1453 (13.7339, 106.5526) -> (18.064, 109.0526)
  line L1454 (18.064, 109.0526) -> (18.064, 114.0526)
  line L1455 (18.064, 114.0526) -> (13.7339, 116.5526)
  line L1456 (24.3941, 116.5526) -> (20.064, 114.0526)
  line L1457 (20.064, 114.0526) -> (20.064, 109.0526)
  line L1458 (20.064, 109.0526) -> (24.3941, 106.5526)
  line L1459 (24.3941, 106.5526) -> (28.7242, 109.0526)
  line L1460 (28.7242, 109.0526) -> (28.7242, 114.0526)
  line L1461 (28.7242, 114.0526) -> (24.3941, 116.5526)
  line L1462 (35.0544, 116.5526) -> (30.7242, 114.0526)
  line L1463 (30.7242, 114.0526) -> (30.7242, 109.0526)
  line L1464 (30.7242, 109.0526) -> (35.0544, 106.5526)
  line L1465 (35.0544, 106.5526) -> (39.3845, 109.0526)
  line L1466 (39.3845, 109.0526) -> (39.3845, 114.0526)
  line L1467 (39.3845, 114.0526) -> (35.0544, 116.5526)
  line L1468 (45.7146, 116.5526) -> (41.3845, 114.0526)
  line L1469 (41.3845, 114.0526) -> (41.3845, 109.0526)
  line L1470 (41.3845, 109.0526) -> (45.7146, 106.5526)
  line L1471 (45.7146, 106.5526) -> (50.0447, 109.0526)
  line L1472 (50.0447, 109.0526) -> (50.0447, 114.0526)
  line L1473 (50.0447, 114.0526) -> (45.7146, 116.5526)
  line L1474 (56.3749, 116.5526) -> (52.0447, 114.0526)
  line L1475 (52.0447, 114.0526) -> (52.0447, 109.0526)
  line L1476 (52.0447, 109.0526) -> (56.3749, 106.5526)
  line L1477 (56.3749, 106.5526) -> (60.705, 109.0526)
  line L1478 (60.705, 109.0526) -> (60.705, 114.0526)
  line L1479 (60.705, 114.0526) -> (56.3749, 116.5526)
  line L1480 (-151.5001, 125.7846) -> (-155.8302, 123.2846)
  line L1481 (-155.8302, 123.2846) -> (-155.8302, 118.2846)
  line L1482 (-155.8302, 118.2846) -> (-151.5001, 115.7846)
  line L1483 (-151.5001, 115.7846) -> (-147.17, 118.2846)
  line L1484 (-147.17, 118.2846) -> (-147.17, 123.2846)
  line L1485 (-147.17, 123.2846) -> (-151.5001, 125.7846)
  line L1486 (-140.8398, 125.7846) -> (-145.17, 123.2846)
  line L1487 (-145.17, 123.2846) -> (-145.17, 118.2846)
  line L1488 (-145.17, 118.2846) -> (-140.8398, 115.7846)
  line L1489 (-140.8398, 115.7846) -> (-136.5097, 118.2846)
  line L1490 (-136.5097, 118.2846) -> (-136.5097, 123.2846)
  line L1491 (-136.5097, 123.2846) -> (-140.8398, 125.7846)
  line L1492 (-130.1796, 125.7846) -> (-134.5097, 123.2846)
  line L1493 (-134.5097, 123.2846) -> (-134.5097, 118.2846)
  line L1494 (-134.5097, 118.2846) -> (-130.1796, 115.7846)
  line L1495 (-130.1796, 115.7846) -> (-125.8494, 118.2846)
  line L1496 (-125.8494, 118.2846) -> (-125.8494, 123.2846)
  line L1497 (-125.8494, 123.2846) -> (-130.1796, 125.7846)
  line L1498 (-119.5193, 125.7846) -> (-123.8494, 123.2846)
  line L1499 (-123.8494, 123.2846) -> (-123.8494, 118.2846)
  line L1500 (-123.8494, 118.2846) -> (-119.5193, 115.7846)
  line L1501 (-119.5193, 115.7846) -> (-115.1892, 118.2846)
  line L1502 (-115.1892, 118.2846) -> (-115.1892, 123.2846)
  line L1503 (-115.1892, 123.2846) -> (-119.5193, 125.7846)
  line L1504 (-108.8591, 125.7846) -> (-113.1892, 123.2846)
  line L1505 (-113.1892, 123.2846) -> (-113.1892, 118.2846)
  line L1506 (-113.1892, 118.2846) -> (-108.8591, 115.7846)
  line L1507 (-108.8591, 115.7846) -> (-104.5289, 118.2846)
  line L1508 (-104.5289, 118.2846) -> (-104.5289, 123.2846)
  line L1509 (-104.5289, 123.2846) -> (-108.8591, 125.7846)
  line L1510 (-98.1988, 125.7846) -> (-102.5289, 123.2846)
  line L1511 (-102.5289, 123.2846) -> (-102.5289, 118.2846)
  line L1512 (-102.5289, 118.2846) -> (-98.1988, 115.7846)
  line L1513 (-98.1988, 115.7846) -> (-93.8687, 118.2846)
  line L1514 (-93.8687, 118.2846) -> (-93.8687, 123.2846)
  line L1515 (-93.8687, 123.2846) -> (-98.1988, 125.7846)
  line L1516 (-87.5386, 125.7846) -> (-91.8687, 123.2846)
  line L1517 (-91.8687, 123.2846) -> (-91.8687, 118.2846)
  line L1518 (-91.8687, 118.2846) -> (-87.5386, 115.7846)
  line L1519 (-87.5386, 115.7846) -> (-83.2084, 118.2846)
  line L1520 (-83.2084, 118.2846) -> (-83.2084, 123.2846)
  line L1521 (-83.2084, 123.2846) -> (-87.5386, 125.7846)
  line L1522 (-76.8783, 125.7846) -> (-81.2084, 123.2846)
  line L1523 (-81.2084, 123.2846) -> (-81.2084, 118.2846)
  line L1524 (-81.2084, 118.2846) -> (-76.8783, 115.7846)
  line L1525 (-76.8783, 115.7846) -> (-72.5482, 118.2846)
  line L1526 (-72.5482, 118.2846) -> (-72.5482, 123.2846)
  line L1527 (-72.5482, 123.2846) -> (-76.8783, 125.7846)
  line L1528 (-66.218, 125.7846) -> (-70.5482, 123.2846)
  line L1529 (-70.5482, 123.2846) -> (-70.5482, 118.2846)
  line L1530 (-70.5482, 118.2846) -> (-66.218, 115.7846)
  line L1531 (-66.218, 115.7846) -> (-61.8879, 118.2846)
  line L1532 (-61.8879, 118.2846) -> (-61.8879, 123.2846)
  line L1533 (-61.8879, 123.2846) -> (-66.218, 125.7846)
  line L1534 (-55.5578, 125.7846) -> (-59.8879, 123.2846)
  line L1535 (-59.8879, 123.2846) -> (-59.8879, 118.2846)
  line L1536 (-59.8879, 118.2846) -> (-55.5578, 115.7846)
  line L1537 (-55.5578, 115.7846) -> (-51.2277, 118.2846)
  line L1538 (-51.2277, 118.2846) -> (-51.2277, 123.2846)
  line L1539 (-51.2277, 123.2846) -> (-55.5578, 125.7846)
  line L1540 (-44.8975, 125.7846) -> (-49.2277, 123.2846)
  line L1541 (-49.2277, 123.2846) -> (-49.2277, 118.2846)
  line L1542 (-49.2277, 118.2846) -> (-44.8975, 115.7846)
  line L1543 (-44.8975, 115.7846) -> (-40.5674, 118.2846)
  line L1544 (-40.5674, 118.2846) -> (-40.5674, 123.2846)
  line L1545 (-40.5674, 123.2846) -> (-44.8975, 125.7846)
  line L1546 (-34.2373, 125.7846) -> (-38.5674, 123.2846)
  line L1547 (-38.5674, 123.2846) -> (-38.5674, 118.2846)
  line L1548 (-38.5674, 118.2846) -> (-34.2373, 115.7846)
  line L1549 (-34.2373, 115.7846) -> (-29.9072, 118.2846)
  line L1550 (-29.9072, 118.2846) -> (-29.9072, 123.2846)
  line L1551 (-29.9072, 123.2846) -> (-34.2373, 125.7846)
  line L1552 (-23.577, 125.7846) -> (-27.9072, 123.2846)
  line L1553 (-27.9072, 123.2846) -> (-27.9072, 118.2846)
  line L1554 (-27.9072, 118.2846) -> (-23.577, 115.7846)
  line L1555 (-23.577, 115.7846) -> (-19.2469, 118.2846)
  line L1556 (-19.2469, 118.2846) -> (-19.2469, 123.2846)
  line L1557 (-19.2469, 123.2846) -> (-23.577, 125.7846)
  line L1558 (-12.9168, 125.7846) -> (-17.2469, 123.2846)
  line L1559 (-17.2469, 123.2846) -> (-17.2469, 118.2846)
  line L1560 (-17.2469, 118.2846) -> (-12.9168, 115.7846)
  line L1561 (-12.9168, 115.7846) -> (-8.5866, 118.2846)
  line L1562 (-8.5866, 118.2846) -> (-8.5866, 123.2846)
  line L1563 (-8.5866, 123.2846) -> (-12.9168, 125.7846)
  line L1564 (-2.2565, 125.7846) -> (-6.5866, 123.2846)
  line L1565 (-6.5866, 123.2846) -> (-6.5866, 118.2846)
  line L1566 (-6.5866, 118.2846) -> (-2.2565, 115.7846)
  line L1567 (-2.2565, 115.7846) -> (2.0736, 118.2846)
  line L1568 (2.0736, 118.2846) -> (2.0736, 123.2846)
  line L1569 (2.0736, 123.2846) -> (-2.2565, 125.7846)
  line L1570 (8.4037, 125.7846) -> (4.0736, 123.2846)
  line L1571 (4.0736, 123.2846) -> (4.0736, 118.2846)
  line L1572 (4.0736, 118.2846) -> (8.4037, 115.7846)
  line L1573 (8.4037, 115.7846) -> (12.7339, 118.2846)
  line L1574 (12.7339, 118.2846) -> (12.7339, 123.2846)
  line L1575 (12.7339, 123.2846) -> (8.4037, 125.7846)
  line L1576 (19.064, 125.7846) -> (14.7339, 123.2846)
  line L1577 (14.7339, 123.2846) -> (14.7339, 118.2846)
  line L1578 (14.7339, 118.2846) -> (19.064, 115.7846)
  line L1579 (19.064, 115.7846) -> (23.3941, 118.2846)
  line L1580 (23.3941, 118.2846) -> (23.3941, 123.2846)
  line L1581 (23.3941, 123.2846) -> (19.064, 125.7846)
  line L1582 (29.7242, 125.7846) -> (25.3941, 123.2846)
  line L1583 (25.3941, 123.2846) -> (25.3941, 118.2846)
  line L1584 (25.3941, 118.2846) -> (29.7242, 115.7846)
  line L1585 (29.7242, 115.7846) -> (34.0544, 118.2846)
  line L1586 (34.0544, 118.2846) -> (34.0544, 123.2846)
  line L1587 (34.0544, 123.2846) -> (29.7242, 125.7846)
  line L1588 (40.3845, 125.7846) -> (36.0544, 123.2846)
  line L1589 (36.0544, 123.2846) -> (36.0544, 118.2846)
  line L1590 (36.0544, 118.2846) -> (40.3845, 115.7846)
  line L1591 (40.3845, 115.7846) -> (44.7146, 118.2846)
  line L1592 (44.7146, 118.2846) -> (44.7146, 123.2846)
  line L1593 (44.7146, 123.2846) -> (40.3845, 125.7846)
  line L1594 (51.0447, 125.7846) -> (46.7146, 123.2846)
  line L1595 (46.7146, 123.2846) -> (46.7146, 118.2846)
  line L1596 (46.7146, 118.2846) -> (51.0447, 115.7846)
  line L1597 (51.0447, 115.7846) -> (55.3749, 118.2846)
  line L1598 (55.3749, 118.2846) -> (55.3749, 123.2846)
  line L1599 (55.3749, 123.2846) -> (51.0447, 125.7846)
  line L1600 (61.705, 125.7846) -> (57.3749, 123.2846)
  line L1601 (57.3749, 123.2846) -> (57.3749, 118.2846)
  line L1602 (57.3749, 118.2846) -> (61.705, 115.7846)
  line L1603 (61.705, 115.7846) -> (66.0351, 118.2846)
  line L1604 (66.0351, 118.2846) -> (66.0351, 123.2846)
  line L1605 (66.0351, 123.2846) -> (61.705, 125.7846)
  line L1606 (-146.17, 135.0167) -> (-150.5001, 132.5167)
  line L1607 (-150.5001, 132.5167) -> (-150.5001, 127.5167)
  line L1608 (-150.5001, 127.5167) -> (-146.17, 125.0167)
  line L1609 (-146.17, 125.0167) -> (-141.8398, 127.5167)
  line L1610 (-141.8398, 127.5167) -> (-141.8398, 132.5167)
  line L1611 (-141.8398, 132.5167) -> (-146.17, 135.0167)
  line L1612 (-135.5097, 135.0167) -> (-139.8398, 132.5167)
  line L1613 (-139.8398, 132.5167) -> (-139.8398, 127.5167)
  line L1614 (-139.8398, 127.5167) -> (-135.5097, 125.0167)
  line L1615 (-135.5097, 125.0167) -> (-131.1796, 127.5167)
  line L1616 (-131.1796, 127.5167) -> (-131.1796, 132.5167)
  line L1617 (-131.1796, 132.5167) -> (-135.5097, 135.0167)
  line L1618 (-124.8494, 135.0167) -> (-129.1796, 132.5167)
  line L1619 (-129.1796, 132.5167) -> (-129.1796, 127.5167)
  line L1620 (-129.1796, 127.5167) -> (-124.8494, 125.0167)
  line L1621 (-124.8494, 125.0167) -> (-120.5193, 127.5167)
  line L1622 (-120.5193, 127.5167) -> (-120.5193, 132.5167)
  line L1623 (-120.5193, 132.5167) -> (-124.8494, 135.0167)
  line L1624 (-114.1892, 135.0167) -> (-118.5193, 132.5167)
  line L1625 (-118.5193, 132.5167) -> (-118.5193, 127.5167)
  line L1626 (-118.5193, 127.5167) -> (-114.1892, 125.0167)
  line L1627 (-114.1892, 125.0167) -> (-109.8591, 127.5167)
  line L1628 (-109.8591, 127.5167) -> (-109.8591, 132.5167)
  line L1629 (-109.8591, 132.5167) -> (-114.1892, 135.0167)
  line L1630 (-103.5289, 135.0167) -> (-107.8591, 132.5167)
  line L1631 (-107.8591, 132.5167) -> (-107.8591, 127.5167)
  line L1632 (-107.8591, 127.5167) -> (-103.5289, 125.0167)
  line L1633 (-103.5289, 125.0167) -> (-99.1988, 127.5167)
  line L1634 (-99.1988, 127.5167) -> (-99.1988, 132.5167)
  line L1635 (-99.1988, 132.5167) -> (-103.5289, 135.0167)
  line L1636 (-92.8687, 135.0167) -> (-97.1988, 132.5167)
  line L1637 (-97.1988, 132.5167) -> (-97.1988, 127.5167)
  line L1638 (-97.1988, 127.5167) -> (-92.8687, 125.0167)
  line L1639 (-92.8687, 125.0167) -> (-88.5386, 127.5167)
  line L1640 (-88.5386, 127.5167) -> (-88.5386, 132.5167)
  line L1641 (-88.5386, 132.5167) -> (-92.8687, 135.0167)
  line L1642 (-82.2084, 135.0167) -> (-86.5386, 132.5167)
  line L1643 (-86.5386, 132.5167) -> (-86.5386, 127.5167)
  line L1644 (-86.5386, 127.5167) -> (-82.2084, 125.0167)
  line L1645 (-82.2084, 125.0167) -> (-77.8783, 127.5167)
  line L1646 (-77.8783, 127.5167) -> (-77.8783, 132.5167)
  line L1647 (-77.8783, 132.5167) -> (-82.2084, 135.0167)
  line L1648 (-71.5482, 135.0167) -> (-75.8783, 132.5167)
  line L1649 (-75.8783, 132.5167) -> (-75.8783, 127.5167)
  line L1650 (-75.8783, 127.5167) -> (-71.5482, 125.0167)
  line L1651 (-71.5482, 125.0167) -> (-67.218, 127.5167)
  line L1652 (-67.218, 127.5167) -> (-67.218, 132.5167)
  line L1653 (-67.218, 132.5167) -> (-71.5482, 135.0167)
  line L1654 (-60.8879, 135.0167) -> (-65.218, 132.5167)
  line L1655 (-65.218, 132.5167) -> (-65.218, 127.5167)
  line L1656 (-65.218, 127.5167) -> (-60.8879, 125.0167)
  line L1657 (-60.8879, 125.0167) -> (-56.5578, 127.5167)
  line L1658 (-56.5578, 127.5167) -> (-56.5578, 132.5167)
  line L1659 (-56.5578, 132.5167) -> (-60.8879, 135.0167)
  line L1660 (-50.2277, 135.0167) -> (-54.5578, 132.5167)
  line L1661 (-54.5578, 132.5167) -> (-54.5578, 127.5167)
  line L1662 (-54.5578, 127.5167) -> (-50.2277, 125.0167)
  line L1663 (-50.2277, 125.0167) -> (-45.8975, 127.5167)
  line L1664 (-45.8975, 127.5167) -> (-45.8975, 132.5167)
  line L1665 (-45.8975, 132.5167) -> (-50.2277, 135.0167)
  line L1666 (-39.5674, 135.0167) -> (-43.8975, 132.5167)
  line L1667 (-43.8975, 132.5167) -> (-43.8975, 127.5167)
  line L1668 (-43.8975, 127.5167) -> (-39.5674, 125.0167)
  line L1669 (-39.5674, 125.0167) -> (-35.2373, 127.5167)
  line L1670 (-35.2373, 127.5167) -> (-35.2373, 132.5167)
  line L1671 (-35.2373, 132.5167) -> (-39.5674, 135.0167)
  line L1672 (-28.9072, 135.0167) -> (-33.2373, 132.5167)
  line L1673 (-33.2373, 132.5167) -> (-33.2373, 127.5167)
  line L1674 (-33.2373, 127.5167) -> (-28.9072, 125.0167)
  line L1675 (-28.9072, 125.0167) -> (-24.577, 127.5167)
  line L1676 (-24.577, 127.5167) -> (-24.577, 132.5167)
  line L1677 (-24.577, 132.5167) -> (-28.9072, 135.0167)
  line L1678 (-18.2469, 135.0167) -> (-22.577, 132.5167)
  line L1679 (-22.577, 132.5167) -> (-22.577, 127.5167)
  line L1680 (-22.577, 127.5167) -> (-18.2469, 125.0167)
  line L1681 (-18.2469, 125.0167) -> (-13.9168, 127.5167)
  line L1682 (-13.9168, 127.5167) -> (-13.9168, 132.5167)
  line L1683 (-13.9168, 132.5167) -> (-18.2469, 135.0167)
  line L1684 (-7.5866, 135.0167) -> (-11.9168, 132.5167)
  line L1685 (-11.9168, 132.5167) -> (-11.9168, 127.5167)
  line L1686 (-11.9168, 127.5167) -> (-7.5866, 125.0167)
  line L1687 (-7.5866, 125.0167) -> (-3.2565, 127.5167)
  line L1688 (-3.2565, 127.5167) -> (-3.2565, 132.5167)
  line L1689 (-3.2565, 132.5167) -> (-7.5866, 135.0167)
  line L1690 (3.0736, 135.0167) -> (-1.2565, 132.5167)
  line L1691 (-1.2565, 132.5167) -> (-1.2565, 127.5167)
  line L1692 (-1.2565, 127.5167) -> (3.0736, 125.0167)
  line L1693 (3.0736, 125.0167) -> (7.4037, 127.5167)
  line L1694 (7.4037, 127.5167) -> (7.4037, 132.5167)
  line L1695 (7.4037, 132.5167) -> (3.0736, 135.0167)
  line L1696 (13.7339, 135.0167) -> (9.4037, 132.5167)
  line L1697 (9.4037, 132.5167) -> (9.4037, 127.5167)
  line L1698 (9.4037, 127.5167) -> (13.7339, 125.0167)
  line L1699 (13.7339, 125.0167) -> (18.064, 127.5167)
  line L1700 (18.064, 127.5167) -> (18.064, 132.5167)
  line L1701 (18.064, 132.5167) -> (13.7339, 135.0167)
  line L1702 (24.3941, 135.0167) -> (20.064, 132.5167)
  line L1703 (20.064, 132.5167) -> (20.064, 127.5167)
  line L1704 (20.064, 127.5167) -> (24.3941, 125.0167)
  line L1705 (24.3941, 125.0167) -> (28.7242, 127.5167)
  line L1706 (28.7242, 127.5167) -> (28.7242, 132.5167)
  line L1707 (28.7242, 132.5167) -> (24.3941, 135.0167)
  line L1708 (35.0544, 135.0167) -> (30.7242, 132.5167)
  line L1709 (30.7242, 132.5167) -> (30.7242, 127.5167)
  line L1710 (30.7242, 127.5167) -> (35.0544, 125.0167)
  line L1711 (35.0544, 125.0167) -> (39.3845, 127.5167)
  line L1712 (39.3845, 127.5167) -> (39.3845, 132.5167)
  line L1713 (39.3845, 132.5167) -> (35.0544, 135.0167)
  line L1714 (45.7146, 135.0167) -> (41.3845, 132.5167)
  line L1715 (41.3845, 132.5167) -> (41.3845, 127.5167)
  line L1716 (41.3845, 127.5167) -> (45.7146, 125.0167)
  line L1717 (45.7146, 125.0167) -> (50.0447, 127.5167)
  line L1718 (50.0447, 127.5167) -> (50.0447, 132.5167)
  line L1719 (50.0447, 132.5167) -> (45.7146, 135.0167)
  line L1720 (56.3749, 135.0167) -> (52.0447, 132.5167)
  line L1721 (52.0447, 132.5167) -> (52.0447, 127.5167)
  line L1722 (52.0447, 127.5167) -> (56.3749, 125.0167)
  line L1723 (56.3749, 125.0167) -> (60.705, 127.5167)
  line L1724 (60.705, 127.5167) -> (60.705, 132.5167)
  line L1725 (60.705, 132.5167) -> (56.3749, 135.0167)
  line L1726 (-151.5001, 144.2487) -> (-155.8302, 141.7487)
  line L1727 (-155.8302, 141.7487) -> (-155.8302, 136.7487)
  line L1728 (-155.8302, 136.7487) -> (-151.5001, 134.2487)
  line L1729 (-151.5001, 134.2487) -> (-147.17, 136.7487)
  line L1730 (-147.17, 136.7487) -> (-147.17, 141.7487)
  line L1731 (-147.17, 141.7487) -> (-151.5001, 144.2487)
  line L1732 (-140.8398, 144.2487) -> (-145.17, 141.7487)
  line L1733 (-145.17, 141.7487) -> (-145.17, 136.7487)
  line L1734 (-145.17, 136.7487) -> (-140.8398, 134.2487)
  line L1735 (-140.8398, 134.2487) -> (-136.5097, 136.7487)
  line L1736 (-136.5097, 136.7487) -> (-136.5097, 141.7487)
  line L1737 (-136.5097, 141.7487) -> (-140.8398, 144.2487)
  line L1738 (-130.1796, 144.2487) -> (-134.5097, 141.7487)
  line L1739 (-134.5097, 141.7487) -> (-134.5097, 136.7487)
  line L1740 (-134.5097, 136.7487) -> (-130.1796, 134.2487)
  line L1741 (-130.1796, 134.2487) -> (-125.8494, 136.7487)
  line L1742 (-125.8494, 136.7487) -> (-125.8494, 141.7487)
  line L1743 (-125.8494, 141.7487) -> (-130.1796, 144.2487)
  line L1744 (-119.5193, 144.2487) -> (-123.8494, 141.7487)
  line L1745 (-123.8494, 141.7487) -> (-123.8494, 136.7487)
  line L1746 (-123.8494, 136.7487) -> (-119.5193, 134.2487)
  line L1747 (-119.5193, 134.2487) -> (-115.1892, 136.7487)
  line L1748 (-115.1892, 136.7487) -> (-115.1892, 141.7487)
  line L1749 (-115.1892, 141.7487) -> (-119.5193, 144.2487)
  line L1750 (-108.8591, 144.2487) -> (-113.1892, 141.7487)
  line L1751 (-113.1892, 141.7487) -> (-113.1892, 136.7487)
  line L1752 (-113.1892, 136.7487) -> (-108.8591, 134.2487)
  line L1753 (-108.8591, 134.2487) -> (-104.5289, 136.7487)
  line L1754 (-104.5289, 136.7487) -> (-104.5289, 141.7487)
  line L1755 (-104.5289, 141.7487) -> (-108.8591, 144.2487)
  line L1756 (-98.1988, 144.2487) -> (-102.5289, 141.7487)
  line L1757 (-102.5289, 141.7487) -> (-102.5289, 136.7487)
  line L1758 (-102.5289, 136.7487) -> (-98.1988, 134.2487)
  line L1759 (-98.1988, 134.2487) -> (-93.8687, 136.7487)
  line L1760 (-93.8687, 136.7487) -> (-93.8687, 141.7487)
  line L1761 (-93.8687, 141.7487) -> (-98.1988, 144.2487)
  line L1762 (-87.5386, 144.2487) -> (-91.8687, 141.7487)
  line L1763 (-91.8687, 141.7487) -> (-91.8687, 136.7487)
  line L1764 (-91.8687, 136.7487) -> (-87.5386, 134.2487)
  line L1765 (-87.5386, 134.2487) -> (-83.2084, 136.7487)
  line L1766 (-83.2084, 136.7487) -> (-83.2084, 141.7487)
  line L1767 (-83.2084, 141.7487) -> (-87.5386, 144.2487)
  line L1768 (-76.8783, 144.2487) -> (-81.2084, 141.7487)
  line L1769 (-81.2084, 141.7487) -> (-81.2084, 136.7487)
  line L1770 (-81.2084, 136.7487) -> (-76.8783, 134.2487)
  line L1771 (-76.8783, 134.2487) -> (-72.5482, 136.7487)
  line L1772 (-72.5482, 136.7487) -> (-72.5482, 141.7487)
  line L1773 (-72.5482, 141.7487) -> (-76.8783, 144.2487)
  line L1774 (-66.218, 144.2487) -> (-70.5482, 141.7487)
  line L1775 (-70.5482, 141.7487) -> (-70.5482, 136.7487)
  line L1776 (-70.5482, 136.7487) -> (-66.218, 134.2487)
  line L1777 (-66.218, 134.2487) -> (-61.8879, 136.7487)
  line L1778 (-61.8879, 136.7487) -> (-61.8879, 141.7487)
  line L1779 (-61.8879, 141.7487) -> (-66.218, 144.2487)
  line L1780 (-55.5578, 144.2487) -> (-59.8879, 141.7487)
  line L1781 (-59.8879, 141.7487) -> (-59.8879, 136.7487)
  line L1782 (-59.8879, 136.7487) -> (-55.5578, 134.2487)
  line L1783 (-55.5578, 134.2487) -> (-51.2277, 136.7487)
  line L1784 (-51.2277, 136.7487) -> (-51.2277, 141.7487)
  line L1785 (-51.2277, 141.7487) -> (-55.5578, 144.2487)
  line L1786 (-44.8975, 144.2487) -> (-49.2277, 141.7487)
  line L1787 (-49.2277, 141.7487) -> (-49.2277, 136.7487)
  line L1788 (-49.2277, 136.7487) -> (-44.8975, 134.2487)
  line L1789 (-44.8975, 134.2487) -> (-40.5674, 136.7487)
  line L1790 (-40.5674, 136.7487) -> (-40.5674, 141.7487)
  line L1791 (-40.5674, 141.7487) -> (-44.8975, 144.2487)
  line L1792 (-34.2373, 144.2487) -> (-38.5674, 141.7487)
  line L1793 (-38.5674, 141.7487) -> (-38.5674, 136.7487)
  line L1794 (-38.5674, 136.7487) -> (-34.2373, 134.2487)
  line L1795 (-34.2373, 134.2487) -> (-29.9072, 136.7487)
  line L1796 (-29.9072, 136.7487) -> (-29.9072, 141.7487)
  line L1797 (-29.9072, 141.7487) -> (-34.2373, 144.2487)
  line L1798 (-23.577, 144.2487) -> (-27.9072, 141.7487)
  line L1799 (-27.9072, 141.7487) -> (-27.9072, 136.7487)
  line L1800 (-27.9072, 136.7487) -> (-23.577, 134.2487)
  line L1801 (-23.577, 134.2487) -> (-19.2469, 136.7487)
  line L1802 (-19.2469, 136.7487) -> (-19.2469, 141.7487)
  line L1803 (-19.2469, 141.7487) -> (-23.577, 144.2487)
  line L1804 (-12.9168, 144.2487) -> (-17.2469, 141.7487)
  line L1805 (-17.2469, 141.7487) -> (-17.2469, 136.7487)
  line L1806 (-17.2469, 136.7487) -> (-12.9168, 134.2487)
  line L1807 (-12.9168, 134.2487) -> (-8.5866, 136.7487)
  line L1808 (-8.5866, 136.7487) -> (-8.5866, 141.7487)
  line L1809 (-8.5866, 141.7487) -> (-12.9168, 144.2487)
  line L1810 (-2.2565, 144.2487) -> (-6.5866, 141.7487)
  line L1811 (-6.5866, 141.7487) -> (-6.5866, 136.7487)
  line L1812 (-6.5866, 136.7487) -> (-2.2565, 134.2487)
  line L1813 (-2.2565, 134.2487) -> (2.0736, 136.7487)
  line L1814 (2.0736, 136.7487) -> (2.0736, 141.7487)
  line L1815 (2.0736, 141.7487) -> (-2.2565, 144.2487)
  line L1816 (8.4037, 144.2487) -> (4.0736, 141.7487)
  line L1817 (4.0736, 141.7487) -> (4.0736, 136.7487)